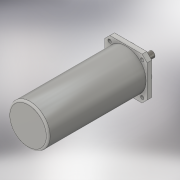
# Autodesk Inventor part: Nanotec-DH052-120E-4N02-Servo
Saved by Autodesk Inventor 2016 (Build 200138000, 138)
## iProperties
Created: 2015-05-16
Part Number: Nanotec-DH052-120E-4N02-Servo
Material: Generic
Document SubType Name: Modeling
Designer: as
Density: 1 g/cm^3
Appearance: Default
Mass: 290.489 g
Surface Area: 286.249 cm^2
Volume: 290.489 cm^3
Author: as
Autodesk Inventor part; units mm, degrees
ref_plane "YZ Plane" through (0, 0, 0) normal (1, 0, 0) x (0, 1, 0)
ref_plane "XZ Plane" through (0, 0, 0) normal (0, 1, 0) x (-1, 0, 0)
ref_plane "XY Plane" through (0, 0, 0) normal (0, 0, 1) x (1, 0, 0)
sketch "Sketch1" plane through (0, 0, 0) normal (0, 1, 0) x (-1, 0, 0)
  line L0 (27.25, 27.25) -> (-27.25, 27.25)
  line L1 (-27.25, 27.25) -> (-27.25, -27.25)
  line L2 (-27.25, -27.25) -> (27.25, -27.25)
  line L3 (27.25, -27.25) -> (27.25, 27.25)
  line L4 (27.25, 27.25) -> (-27.25, -27.25) construction
  line L5 (-27.25, 27.25) -> (27.25, -27.25) construction
  line L6 (21, 21) -> (-21, 21)
  line L7 (-21, 21) -> (-21, -21)
  line L8 (-21, -21) -> (21, -21)
  line L9 (21, -21) -> (21, 21)
  line L10 (21, 21) -> (-21, -21) construction
  line L11 (-21, 21) -> (21, -21) construction
  point P0 (0, 0)
  dimension "d0" = 54.5
  dimension "d1" = 54.5
  dimension "d2" = 42
  dimension "d3" = 42
  constraints: 24 end point, 4 coincident, 4 midpoint, 4 parallel, 2 horizontal, 2 perpendicular
  measures "d0" distance of L2.end L1.end
  measures "d1" distance of L0.end L1.end
  measures "d2" distance of L8.end L7.end
  measures "d3" distance of L6.end L7.end
extrude "Extrusion1" add sketch "Sketch1" along normal blind 6 contours L3 L2 L1 L0 | L9 L8 L7 L6
sketch "Sketch2" plane through (0, 6, 0) normal (0, 1, 0) x (1, 0, 0)
  circle A0 centre (0, 0) radius 25
  dimension "d7" = 50
  constraints: 1 centre point, 1 coincident
  measures "d7" diameter of A0
extrude "Extrusion2" add sketch "Sketch2" along normal blind 2.5
sketch "Sketch3" plane through (0, 0, 0) normal (0, -1, 0) x (1, 0, 0)
  circle A0 centre (0, 0) radius 26
  dimension "d10" = 52
  constraints: 1 centre point, 1 coincident
  measures "d10" diameter of A0
extrude "Extrusion3" add sketch "Sketch3" along normal blind 126
fillet "Fillet1" radius 2.5 1 edges at (-26, -126, 0)
hole "Hole1" at (21, 0, -21) at (21, 0, 21) at (-21, 0, -21) at (-21, 0, 21) direction (0, 1, 0) diameter 4.4 end through all
sketch "Sketch4" plane through (0, 8.5, 0) normal (0, 1, 0) x (1, 0, 0)
  circle A0 centre (0, 0) radius 4
  dimension "d22" = 8
  constraints: 1 centre point, 1 coincident
  measures "d22" diameter of A0
extrude "Extrusion4" add sketch "Sketch4" along normal blind 25
chamfer "Chamfer1" distance 6.5 angle 45 4 edges at (27.25, 3, 27.25) (27.25, 3, -27.25) (-27.25, 3, -27.25) (-27.25, 3, 27.25)
equation "\"d1\" = d0"
equation "\"d3\" = d2"
body "Solid1"
